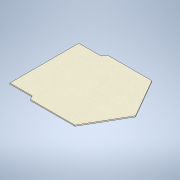
# Autodesk Inventor part: PlayerTacticalMats_All
Saved by Autodesk Inventor 2021 (Build 250183000, 183)
## iProperties
Created: 2023-03-16
Part Number: PlayerTacticalMats_All
Material: Paper
Document SubType Name: Modeling
Designer: Bradley
Density: 0.93 g/cm^3
Appearance: Cardboard - Chipboard
Author: Bradley
Autodesk Inventor part; units mm, degrees
ref_plane "YZ Plane" through (0, 0, 0) normal (1, 0, 0) x (0, 1, 0)
ref_plane "XZ Plane" through (0, 0, 0) normal (0, 1, 0) x (-1, 0, 0)
ref_plane "XY Plane" through (0, 0, 0) normal (0, 0, 1) x (1, 0, 0)
sketch "Sketch1" plane through (0, 0, 0) normal (0, 1, 0) x (-1, 0, 0)
  line L0 (-110.2739, 0) -> (-55.137, 95.5)
  line L1 (-55.137, 95.5) -> (55.137, 95.5)
  line L2 (55.137, 95.5) -> (110.2739, 0)
  line L3 (110.2739, 0) -> (55.137, -95.5)
  line L4 (55.137, -95.5) -> (-55.137, -95.5)
  line L5 (-55.137, -95.5) -> (-110.2739, 0)
  line L6 (60.9105, -85.5) -> (116, -85.5)
  line L7 (116, -85.5) -> (116, 85.5)
  line L8 (116, 85.5) -> (60.9105, 85.5)
  point P0 (0, 0)
  point P1 (0, 0)
  point P2 (116, 0)
  dimension "d5" = 191
  dimension "d6" = 171
  dimension "d7" = 116
  constraints: 18 end point, 2 horizontal, 2 perpendicular, 2 point on line, 1 coincident, 1 horizontal alignment, 1 midpoint, 13 other
  measures "d5" distance between parallel lines of L1 L4
  measures "d6" distance of L6.end L7.end
  measures "d7" distance from line of point (0, 0) L7
extrude "Extrusion1" add sketch "Sketch1" along normal mid plane 2.55
body "Solid1"
